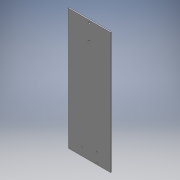
# Autodesk Inventor part: Force_Arm_board
Saved by Autodesk Inventor 2016 (Build 200138000, 138)
## iProperties
Created: 2016-11-14
Part Number: Force_Arm_board
Material: 一般
Document SubType Name: Modeling
Designer: 宏太
Density: 1 g/cm^3
Appearance: 既定
Author: 宏太
Autodesk Inventor part; units mm, degrees
ref_plane "YZ Plane" through (0, 0, 0) normal (1, 0, 0) x (0, 1, 0)
ref_plane "XZ Plane" through (0, 0, 0) normal (0, 1, 0) x (-1, 0, 0)
ref_plane "XY Plane" through (0, 0, 0) normal (0, 0, 1) x (1, 0, 0)
sketch "スケッチ1" plane through (0, 0, 0) normal (0, 1, 0) x (-1, 0, 0)
  line L0 (0, 0) -> (80, 0)
  line L1 (80, 0) -> (80, 230)
  line L2 (80, 230) -> (0, 230)
  line L3 (0, 230) -> (0, 0)
  dimension "d0" = 80
  dimension "d1" = 230
  constraints: 8 end point, 2 parallel, 1 horizontal, 1 perpendicular
  measures "d0" distance of L2.end L1.end
  measures "d1" distance of L1.end L0.end
extrude "押し出し1" add sketch "スケッチ1" along normal blind 2
sketch "スケッチ2" plane through (0, 2, 0) normal (0, 1, 0) x (1, 0, 0)
  line L0 (0, 0) -> (-80, 0) projected
  line L1 (0, -230) -> (0, 0) projected
  circle A0 centre (-40, -225) radius 2
  line L2 (-80, -230) -> (0, -230) projected
  circle A1 centre (-40, -195) radius 2
  circle A2 centre (-26.5, -2) radius 1
  circle A3 centre (-26.5, -20.5) radius 1
  circle A4 centre (-53.5, -15.5) radius 1
  dimension "d9" = 4
  dimension "d10" = 5
  dimension "d11" = 40
  dimension "d12" = 4
  dimension "d13" = 30
  dimension "d16" = 2
  dimension "d17" = 2
  dimension "d18" = 2
  dimension "d19" = 228
  dimension "d20" = 209.5
  dimension "d21" = 214.5
  dimension "d22" = 53.5
  dimension "d23" = 26.5
  dimension "d24" = 26.5
  constraints: 5 centre point
  measures "d9" diameter of A0
  measures "d10" distance from line of L2 A0.centre
  measures "d11" distance from line of L1 A0.centre
  measures "d12" diameter of A1
  measures "d13" distance of A1.centre A0.centre
  measures "d16" diameter of A2
  measures "d17" diameter of A3
  measures "d18" diameter of A4
  measures "d19" distance from line of L2 A2.centre
  measures "d20" distance from line of L2 A3.centre
  measures "d21" distance from line of L2 A4.centre
  measures "d22" distance from line of L1 A4.centre
  measures "d23" distance from line of L1 A3.centre
  measures "d24" distance from line of L1 A2.centre
extrude "押し出し3" cut sketch "スケッチ2" against normal blind 10
